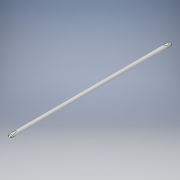
# Autodesk Inventor part: Straight connector
Saved by Autodesk Inventor 2018 (Build 220112000, 112)
## iProperties
Created: 2019-05-31
Part Number: Straight connector
Material: Generic
Document SubType Name: Modeling
Designer: ch1180245
Density: 1 g/cm^3
Appearance: Default
Author: ch1180245
Autodesk Inventor part; units mm, degrees
ref_plane "XZ Plane" through (0, 0, 0) normal (0, 1, 0) x (-1, 0, 0)
sketch "Sketch1" plane through (0, 0, 0) normal (0, 1, 0) x (-1, 0, 0)
  circle A0 centre (0, 0) radius 5
  dimension "d0" = 10
  constraints: 1 centre point, 1 coincident
  measures "d0" diameter of A0
extrude "Extrusion1" add sketch "Sketch1" along normal blind 500
ref_plane "Work Plane1" through (5, 0, 0) normal (1, 0, 0) x (0, 1, 0)
sketch "Sketch2" plane through (5, 0, 0) normal (1, 0, 0) x (0, 1, 0)
  line L0 (500, -5) -> (500, 5) projected
  line L1 (0, 5) -> (0, -5) projected
  line L2 (0, 5) -> (500, 5) projected
  line L3 (0, -5) -> (500, -5) projected
  line L4 (0, 0) -> (0, 1.5)
  line L5 (0, 5) -> (0, -5) projected
  line L6 (0, 0) -> (0, -1.5)
  line L7 (-100, 0) -> (600, 0) projected
  line L8 (0, 1.5) -> (20, 5)
  line L9 (20, 5) -> (20, -5)
  line L10 (20, -5) -> (0, -1.5)
  dimension "d4" = 1.5
  dimension "d5" = 1.5
  dimension "d6" = 20
  constraints: 10 end point, 4 point on line, 1 perpendicular
  measures "d4" distance of L4.end L4.start
  measures "d5" distance of L4.start L6.end
  measures "d6" distance of L1.start L8.end
extrude "Extrusion2" cut sketch "Sketch2" against normal blind 500 contours L3 L1 L10 | L8 L1 L2
sketch "Sketch3" plane through (0, 0, 0) normal (0, 0, 1) x (1, 0, 0)
  point P0 (0, 0)
sketch "Sketch4" plane through (0, 0, 0) normal (0, 0, 1) x (1, 0, 0)
  circle A0 centre (0, 4.565) radius 1
  point P0 (0, 0)
  dimension "d9" = 2
  constraints: 1 centre point
  measures "d9" diameter of A0
extrude "Extrusion3" cut sketch "Sketch4" along normal mid plane 500
ref_plane "Work Plane2" through (0, 250, 0) normal (0, -1, 0) x (1, 0, 0)
mirror "Mirror1" about plane through (0, 250, 0) normal (0, -1, 0) of "Extrusion2", "Extrusion3"
body "Solid1"
